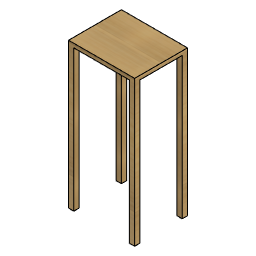
Table (Autodesk Fusion 360 design; units mm, degrees)
Autodesk Fusion 360 part; units mm, degrees
box "PrimitivaParallelepipedo1" add length 400 width 500 height 30 placed x (0, 1, 0) y (-1, 0, 0) z (0, 0, 1) at (500, 0, 0)
sketch "Schizzo2" plane through (0, 0, 0) normal (0, 0, -1) x (1, 0, 0)
  line L0 (0, -400) -> (500, -400)
  line L1 (500, -400) -> (500, 0)
  line L2 (500, 0) -> (0, 0)
  line L3 (0, 0) -> (0, -400)
  line L4 (0, 0) -> (40, 0)
  line L5 (40, 0) -> (40, -40)
  line L6 (40, -40) -> (0, -40)
  line L7 (0, -40) -> (0, 0)
  line L8 (500, 0) -> (460, 0)
  line L9 (460, 0) -> (460, -40)
  line L10 (460, -40) -> (500, -40)
  line L11 (500, -40) -> (500, 0)
  line L12 (500, -400) -> (460, -400)
  line L13 (460, -400) -> (460, -360)
  line L14 (460, -360) -> (500, -360)
  line L15 (500, -360) -> (500, -400)
  line L16 (0, -400) -> (40, -400)
  line L17 (40, -400) -> (40, -360)
  line L18 (40, -360) -> (0, -360)
  line L19 (0, -360) -> (0, -400)
  dimension "d6" = 40
  dimension "d7" = 40
  dimension "d8" = 40
  dimension "d9" = 40
  constraint horizontal L4
  constraint vertical L5
  constraint horizontal L6
  constraint vertical L7
  constraint coincident L2.end L3.start
  constraint horizontal L8
  constraint vertical L9
  constraint horizontal L10
  constraint vertical L11
  constraint coincident L1.end L2.start
  constraint horizontal L12
  constraint vertical L13
  constraint horizontal L14
  constraint vertical L15
  constraint coincident L0.end L1.start
  constraint horizontal L16
  constraint vertical L17
  constraint horizontal L18
  constraint vertical L19
  constraint coincident L0.start L3.end
  constraint equal L10 L14
  constraint equal L13 L14
  constraint equal L17 L18
  constraint equal L6 L17
  measures "d6" distance of L2.end L4.end
  measures "d7" distance of L2.end L6.end
  measures "d8" distance of L1.end L8.end
  measures "d9" distance of L1.end L10.end
extrude "Estrusione1" add sketch "Schizzo2" along normal blind 1070 contours L0 L3 L16 L17 L18 L19 | L0 L1 L12 L13 L14 L15 | L2 L3 L4 L5 L6 L7 | L1 L2 L8 L9 L10 L11
component "Component" placed x (1, 0, 0) y (0, 1, 0) z (0, 0, 1) at (0, 0, 0)
